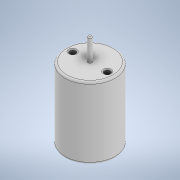
# Autodesk Inventor part: RS-385 Dc Electric Motor
Saved by Autodesk Inventor 2020.2 (Build 242310000, 310)
## iProperties
Created: 2020-04-11
Part Number: RS-385 Dc Electric Motor
Material: Generic
Document SubType Name: Modeling
Designer: Josiah
Density: 1 g/cm^3
Appearance: Default
Author: Josiah
Autodesk Inventor part; units mm, degrees
ref_plane "YZ Plane" through (0, 0, 0) normal (1, 0, 0) x (0, 1, 0)
ref_plane "XZ Plane" through (0, 0, 0) normal (0, 1, 0) x (-1, 0, 0)
ref_plane "XY Plane" through (0, 0, 0) normal (0, 0, 1) x (1, 0, 0)
sketch "Sketch2" plane through (0, 0, 0) normal (0, 1, 0) x (-1, 0, 0)
  circle A0 centre (0, 0) radius 12.3
  dimension "d1" = 24.6
  constraints: 1 centre point, 1 coincident
  measures "d1" diameter of A0
extrude "Extrusion1" add sketch "Sketch2" along normal blind 35.2
sketch "Sketch3" plane through (0, 35.2, 0) normal (0, 1, 0) x (1, 0, 0)
  circle A0 centre (0, 0) radius 1
  dimension "d4" = 2
  constraints: 1 centre point, 1 coincident
  measures "d4" diameter of A0
extrude "Extrusion2" add sketch "Sketch3" along normal blind 11
sketch "Sketch4" plane through (0, 35.2, 0) normal (0, 1, 0) x (1, 0, 0)
  circle A0 centre (-8.5, 0) radius 1.5
  circle A1 centre (8.5, 0) radius 1.5
  point P0 (0, 0)
  dimension "d7" = 3
  dimension "d9" = 8.5
  dimension "d13" = 360
  constraints: 2 centre point, 5 other
  measures "d7" diameter of A0
  measures "d9" distance of point (0, 0) A0.centre
extrude "Extrusion3" cut sketch "Sketch4" against normal blind 17
thread "Thread1" size "M3x0.5" class "6H" standard "ANSI Metric M Profile" full length
thread "Thread2" size "M3x0.5" class "6H" standard "ANSI Metric M Profile" full length
fillet "Fillet1" radius 1 2 edges at (12.3, 35.2, 0) (12.3, 0, 0)
fillet "Fillet1" radius 0.5 3 edges at (-10, 35.2, 0) (7, 35.2, 0) (-1, 46.2, 0)
body "Solid1"
